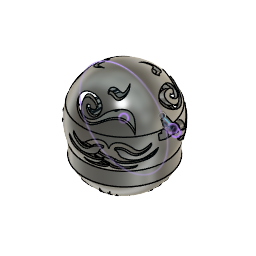
board+case (Autodesk Fusion 360 design; units mm, degrees)
part number: 2025-12-10-14-29-19-279
part number: 2025-12-10-14-29-30-996
part number: 2025-12-10-16-31-34-686
part number: 2025-12-10-16-59-24-375
part number: 2025-12-10-23-41-42-492
part number: 2025-12-11-01-50-10-497
part number: 2025-12-11-01-57-33-360
part number: 2025-12-11-03-29-09-115
Autodesk Fusion 360 part; units mm, degrees
(part 1 of 2)
sketch "Sketch1" plane through (0, 0, 0) normal (0, 0, 1) x (1, 0, 0) in component "base"
  circle A0 centre (0, 0) radius 0.45
  circle A1 centre (2.54, 0) radius 0.45
  circle A2 centre (5.08, 0) radius 0.45
  circle A3 centre (7.62, 0) radius 0.45
  circle A4 centre (10.16, 0) radius 0.45
  circle A5 centre (12.7, 0) radius 0.45
  circle A6 centre (15.24, 0) radius 0.45
  circle A7 centre (17.78, 0) radius 0.45
  circle A8 centre (20.32, 0) radius 0.45
  circle A9 centre (22.86, 0) radius 0.45
  circle A10 centre (25.4, 0) radius 0.45
  circle A11 centre (27.94, 0) radius 0.45
  circle A12 centre (30.48, 0) radius 0.45
  circle A13 centre (33.02, 0) radius 0.45
  circle A14 centre (35.56, 0) radius 0.45
  circle A15 centre (0, 2.54) radius 0.45
  circle A16 centre (2.54, 2.54) radius 0.45
  circle A17 centre (5.08, 2.54) radius 0.45
  circle A18 centre (7.62, 2.54) radius 0.45
  circle A19 centre (10.16, 2.54) radius 0.45
  circle A20 centre (12.7, 2.54) radius 0.45
  circle A21 centre (15.24, 2.54) radius 0.45
  circle A22 centre (17.78, 2.54) radius 0.45
  circle A23 centre (20.32, 2.54) radius 0.45
  circle A24 centre (22.86, 2.54) radius 0.45
  circle A25 centre (25.4, 2.54) radius 0.45
  circle A26 centre (27.94, 2.54) radius 0.45
  circle A27 centre (30.48, 2.54) radius 0.45
  circle A28 centre (33.02, 2.54) radius 0.45
  circle A29 centre (35.56, 2.54) radius 0.45
  circle A30 centre (0, 5.08) radius 0.45
  circle A31 centre (2.54, 5.08) radius 0.45
  circle A32 centre (5.08, 5.08) radius 0.45
  circle A33 centre (7.62, 5.08) radius 0.45
  circle A34 centre (10.16, 5.08) radius 0.45
  circle A35 centre (12.7, 5.08) radius 0.45
  circle A36 centre (15.24, 5.08) radius 0.45
  circle A37 centre (17.78, 5.08) radius 0.45
  circle A38 centre (20.32, 5.08) radius 0.45
  circle A39 centre (22.86, 5.08) radius 0.45
  circle A40 centre (25.4, 5.08) radius 0.45
  circle A41 centre (27.94, 5.08) radius 0.45
  circle A42 centre (30.48, 5.08) radius 0.45
  circle A43 centre (33.02, 5.08) radius 0.45
  circle A44 centre (35.56, 5.08) radius 0.45
  circle A45 centre (0, 7.62) radius 0.45
  circle A46 centre (2.54, 7.62) radius 0.45
  circle A47 centre (5.08, 7.62) radius 0.45
  circle A48 centre (7.62, 7.62) radius 0.45
  circle A49 centre (10.16, 7.62) radius 0.45
  circle A50 centre (12.7, 7.62) radius 0.45
  circle A51 centre (15.24, 7.62) radius 0.45
  circle A52 centre (17.78, 7.62) radius 0.45
  circle A53 centre (20.32, 7.62) radius 0.45
  circle A54 centre (22.86, 7.62) radius 0.45
  circle A55 centre (25.4, 7.62) radius 0.45
  circle A56 centre (27.94, 7.62) radius 0.45
  circle A57 centre (30.48, 7.62) radius 0.45
  circle A58 centre (33.02, 7.62) radius 0.45
  circle A59 centre (35.56, 7.62) radius 0.45
  circle A60 centre (0, 10.16) radius 0.45
  circle A61 centre (2.54, 10.16) radius 0.45
  circle A62 centre (5.08, 10.16) radius 0.45
  circle A63 centre (7.62, 10.16) radius 0.45
  circle A64 centre (10.16, 10.16) radius 0.45
  circle A65 centre (12.7, 10.16) radius 0.45
  circle A66 centre (15.24, 10.16) radius 0.45
  circle A67 centre (17.78, 10.16) radius 0.45
  circle A68 centre (20.32, 10.16) radius 0.45
  circle A69 centre (22.86, 10.16) radius 0.45
  circle A70 centre (25.4, 10.16) radius 0.45
  circle A71 centre (27.94, 10.16) radius 0.45
  circle A72 centre (30.48, 10.16) radius 0.45
  circle A73 centre (33.02, 10.16) radius 0.45
  circle A74 centre (35.56, 10.16) radius 0.45
  circle A75 centre (0, 12.7) radius 0.45
  circle A76 centre (2.54, 12.7) radius 0.45
  circle A77 centre (5.08, 12.7) radius 0.45
  circle A78 centre (7.62, 12.7) radius 0.45
  circle A79 centre (10.16, 12.7) radius 0.45
  circle A80 centre (12.7, 12.7) radius 0.45
  circle A81 centre (15.24, 12.7) radius 0.45
  circle A82 centre (17.78, 12.7) radius 0.45
  circle A83 centre (20.32, 12.7) radius 0.45
  circle A84 centre (22.86, 12.7) radius 0.45
  circle A85 centre (25.4, 12.7) radius 0.45
  circle A86 centre (27.94, 12.7) radius 0.45
  circle A87 centre (30.48, 12.7) radius 0.45
  circle A88 centre (33.02, 12.7) radius 0.45
  circle A89 centre (35.56, 12.7) radius 0.45
  circle A90 centre (0, 15.24) radius 0.45
  circle A91 centre (2.54, 15.24) radius 0.45
  circle A92 centre (5.08, 15.24) radius 0.45
  circle A93 centre (7.62, 15.24) radius 0.45
  circle A94 centre (10.16, 15.24) radius 0.45
  circle A95 centre (12.7, 15.24) radius 0.45
  circle A96 centre (15.24, 15.24) radius 0.45
  circle A97 centre (17.78, 15.24) radius 0.45
  circle A98 centre (20.32, 15.24) radius 0.45
  circle A99 centre (22.86, 15.24) radius 0.45
  circle A100 centre (25.4, 15.24) radius 0.45
  circle A101 centre (27.94, 15.24) radius 0.45
  circle A102 centre (30.48, 15.24) radius 0.45
  circle A103 centre (33.02, 15.24) radius 0.45
  circle A104 centre (35.56, 15.24) radius 0.45
  circle A105 centre (0, 17.78) radius 0.45
  circle A106 centre (2.54, 17.78) radius 0.45
  circle A107 centre (5.08, 17.78) radius 0.45
  circle A108 centre (7.62, 17.78) radius 0.45
  circle A109 centre (10.16, 17.78) radius 0.45
  circle A110 centre (12.7, 17.78) radius 0.45
  circle A111 centre (15.24, 17.78) radius 0.45
  circle A112 centre (17.78, 17.78) radius 0.45
  circle A113 centre (20.32, 17.78) radius 0.45
  circle A114 centre (22.86, 17.78) radius 0.45
  circle A115 centre (25.4, 17.78) radius 0.45
  circle A116 centre (27.94, 17.78) radius 0.45
  circle A117 centre (30.48, 17.78) radius 0.45
  circle A118 centre (33.02, 17.78) radius 0.45
  circle A119 centre (35.56, 17.78) radius 0.45
  circle A120 centre (0, 20.32) radius 0.45
  circle A121 centre (2.54, 20.32) radius 0.45
  circle A122 centre (5.08, 20.32) radius 0.45
  circle A123 centre (7.62, 20.32) radius 0.45
  circle A124 centre (10.16, 20.32) radius 0.45
  circle A125 centre (12.7, 20.32) radius 0.45
  circle A126 centre (15.24, 20.32) radius 0.45
  circle A127 centre (17.78, 20.32) radius 0.45
  circle A128 centre (20.32, 20.32) radius 0.45
  circle A129 centre (22.86, 20.32) radius 0.45
  circle A130 centre (25.4, 20.32) radius 0.45
  circle A131 centre (27.94, 20.32) radius 0.45
  circle A132 centre (30.48, 20.32) radius 0.45
  circle A133 centre (33.02, 20.32) radius 0.45
  circle A134 centre (35.56, 20.32) radius 0.45
  circle A135 centre (0, 22.86) radius 0.45
  circle A136 centre (2.54, 22.86) radius 0.45
  circle A137 centre (5.08, 22.86) radius 0.45
  circle A138 centre (7.62, 22.86) radius 0.45
  circle A139 centre (10.16, 22.86) radius 0.45
  circle A140 centre (12.7, 22.86) radius 0.45
  circle A141 centre (15.24, 22.86) radius 0.45
  circle A142 centre (17.78, 22.86) radius 0.45
  circle A143 centre (20.32, 22.86) radius 0.45
  circle A144 centre (22.86, 22.86) radius 0.45
  circle A145 centre (25.4, 22.86) radius 0.45
  circle A146 centre (27.94, 22.86) radius 0.45
  circle A147 centre (30.48, 22.86) radius 0.45
  circle A148 centre (33.02, 22.86) radius 0.45
  circle A149 centre (35.56, 22.86) radius 0.45
  circle A150 centre (0, 25.4) radius 0.45
  circle A151 centre (2.54, 25.4) radius 0.45
  circle A152 centre (5.08, 25.4) radius 0.45
  circle A153 centre (7.62, 25.4) radius 0.45
  circle A154 centre (10.16, 25.4) radius 0.45
  circle A155 centre (12.7, 25.4) radius 0.45
  circle A156 centre (15.24, 25.4) radius 0.45
  circle A157 centre (17.78, 25.4) radius 0.45
  circle A158 centre (20.32, 25.4) radius 0.45
  circle A159 centre (22.86, 25.4) radius 0.45
  circle A160 centre (25.4, 25.4) radius 0.45
  circle A161 centre (27.94, 25.4) radius 0.45
  circle A162 centre (30.48, 25.4) radius 0.45
  circle A163 centre (33.02, 25.4) radius 0.45
  circle A164 centre (35.56, 25.4) radius 0.45
  circle A165 centre (0, 27.94) radius 0.45
  circle A166 centre (2.54, 27.94) radius 0.45
  circle A167 centre (5.08, 27.94) radius 0.45
  circle A168 centre (7.62, 27.94) radius 0.45
  circle A169 centre (10.16, 27.94) radius 0.45
  circle A170 centre (12.7, 27.94) radius 0.45
  circle A171 centre (15.24, 27.94) radius 0.45
  circle A172 centre (17.78, 27.94) radius 0.45
  circle A173 centre (20.32, 27.94) radius 0.45
  circle A174 centre (22.86, 27.94) radius 0.45
  circle A175 centre (25.4, 27.94) radius 0.45
  circle A176 centre (27.94, 27.94) radius 0.45
  circle A177 centre (30.48, 27.94) radius 0.45
  circle A178 centre (33.02, 27.94) radius 0.45
  circle A179 centre (35.56, 27.94) radius 0.45
  circle A180 centre (0, 30.48) radius 0.45
  circle A181 centre (2.54, 30.48) radius 0.45
  circle A182 centre (5.08, 30.48) radius 0.45
  circle A183 centre (7.62, 30.48) radius 0.45
  circle A184 centre (10.16, 30.48) radius 0.45
  circle A185 centre (12.7, 30.48) radius 0.45
  circle A186 centre (15.24, 30.48) radius 0.45
  circle A187 centre (17.78, 30.48) radius 0.45
  circle A188 centre (20.32, 30.48) radius 0.45
  circle A189 centre (22.86, 30.48) radius 0.45
  circle A190 centre (25.4, 30.48) radius 0.45
  circle A191 centre (27.94, 30.48) radius 0.45
  circle A192 centre (30.48, 30.48) radius 0.45
  circle A193 centre (33.02, 30.48) radius 0.45
  circle A194 centre (35.56, 30.48) radius 0.45
  circle A195 centre (0, 33.02) radius 0.45
  circle A196 centre (2.54, 33.02) radius 0.45
  circle A197 centre (5.08, 33.02) radius 0.45
  circle A198 centre (7.62, 33.02) radius 0.45
  circle A199 centre (10.16, 33.02) radius 0.45
  circle A200 centre (12.7, 33.02) radius 0.45
  circle A201 centre (15.24, 33.02) radius 0.45
  circle A202 centre (17.78, 33.02) radius 0.45
  circle A203 centre (20.32, 33.02) radius 0.45
  circle A204 centre (22.86, 33.02) radius 0.45
  circle A205 centre (25.4, 33.02) radius 0.45
  circle A206 centre (27.94, 33.02) radius 0.45
  circle A207 centre (30.48, 33.02) radius 0.45
  circle A208 centre (33.02, 33.02) radius 0.45
  circle A209 centre (35.56, 33.02) radius 0.45
  circle A210 centre (0, 35.56) radius 0.45
  circle A211 centre (2.54, 35.56) radius 0.45
  circle A212 centre (5.08, 35.56) radius 0.45
  circle A213 centre (7.62, 35.56) radius 0.45
  circle A214 centre (10.16, 35.56) radius 0.45
  circle A215 centre (12.7, 35.56) radius 0.45
  circle A216 centre (15.24, 35.56) radius 0.45
  circle A217 centre (17.78, 35.56) radius 0.45
  circle A218 centre (20.32, 35.56) radius 0.45
  circle A219 centre (22.86, 35.56) radius 0.45
  circle A220 centre (25.4, 35.56) radius 0.45
  circle A221 centre (27.94, 35.56) radius 0.45
  circle A222 centre (30.48, 35.56) radius 0.45
  circle A223 centre (33.02, 35.56) radius 0.45
  circle A224 centre (35.56, 35.56) radius 0.45
  line L0 (-2, 38) -> (38, 38)
  line L1 (38, 38) -> (38, -2)
  line L2 (38, -2) -> (-2, -2)
  line L3 (-2, -2) -> (-2, 38)
  dimension "d1" = 0.9
  dimension "d4" = 2.54
  dimension "d5" = 2.54
  dimension "d6" = 40
  dimension "d7" = 40
  constraint coincident A0.centre origin
  constraint horizontal L0
  constraint vertical L1
  constraint horizontal L2
  constraint vertical L3
  measures "d1" diameter of A0
  measures "d6" distance of L0.start L0.end
  measures "d7" distance of L0.start L2.end
extrude "Extrude1" add sketch "Sketch1" along normal blind 2 contours A0 | A1 | A2 | A3 | A4 | A5 | A6 | A7 | A8 | A9 | A10 | A11 | A12 | A13 | A14 | A15 | A17 | A18 | A19 | A20 | A21 | A22 | A23 | A24 | A25 | A27 | A28 | A29 | A30 | A31 | A32 | A33 | A34 | A35 | A36 | A37 | A38 | A39 | A40 | A41 | A42 | A43 | A44 | A45 | A46 | A47 | A48 | A49 | A50 | A51 | A52 | A53 | A54 | A55 | A56 | A57 | A58 | A59 | A60 | A61 | A62 | A63 | A64 | A65 | A66 | A67 | A68 | A69 | A70 | A71 | A72 | A73 | A74 | A75 | A76 | A77 | A78 | A79 | A80 | A81 | A82 | A83 | A84 | A85 | A86 | A87 | A88 | A89 | A90 | A91 | A92 | A93 | A94 | A95 | A96 | A97 | A98 | A99 | A100 | A101 | A102 | A103 | A104 | A105 | A106 | A107 | A108 | A109 | A110 | A111 | A112 | A113 | A114 | A115 | A116 | A117 | A118 | A119 | A120 | A121 | A122 | A123 | A124 | A125 | A126 | A127 | A128 | A129 | A130 | A131 | A132 | A133 | A134 | A135 | A136 | A137 | A138 | A139 | A140 | A141 | A142 | A143 | A144 | A145 | A146 | A147 | A148 | A149 | A150 | A151 | A152 | A153 | A154 | A155 | A156 | A157 | A158 | A159 | A160 | A161 | A162 | A163 | A164 | A165 | A167 | A168 | A169 | A170 | A171 | A172 | A173 | A174 | A175 | A177 | A178 | A179 | A180 | A181 | A182 | A183 | A184 | A185 | A186 | A187 | A188 | A189 | A190 | A191 | A192 | A193 | A194 | A195 | A196 | A197 | A198 | A199 | A200 | A201 | A202 | A203 | A204 | A205 | A206 | A207 | A208 | A209 | A210 | A211 | A212 | A213 | A214 | A215 | A216 | A217 | A218 | A219 | A220 | A221 | A222 | A223 | A224 | L0 L1 L2 L3 makes body 1 in component "base"
sketch "Sketch2" plane through (0, 0, 0) normal (0, 0, -1) x (1, 0, 0) in component "base"
  circle A0 centre (2.54, -27.94) radius 0.45
  circle A1 centre (27.94, -2.54) radius 0.45
  circle A2 centre (27.94, -27.94) radius 0.45
  circle A3 centre (2.54, -2.54) radius 0.45
  line L0 (38, 2) -> (-2, 2)
  line L1 (-2, 2) -> (-2, -38)
  line L2 (-2, -38) -> (38, -38)
  line L3 (38, -38) -> (38, 2)
  line L4 (39.5, 3.5) -> (-3.5, 3.5)
  line L5 (-3.5, 3.5) -> (-3.5, -39.5)
  line L6 (-3.5, -39.5) -> (39.5, -39.5)
  line L7 (39.5, -39.5) -> (39.5, 3.5)
  dimension "d10" = 1.5
extrude "Extrude2" add sketch "Sketch2" against normal blind 27 contours L4 L5 L6 L7 bodies 1 in component "base"
sketch "Sketch3" plane through (0, 0, 27) normal (0, 0, 1) x (-1, 0, 0) in component "base"
  line L0 (-38, -38) -> (-38, 2)
  line L1 (-38, 2) -> (2, 2)
  line L2 (2, 2) -> (2, -38)
  line L3 (2, -38) -> (-38, -38)
  line L4 (-39.5, 3.5) -> (-39.5, -39.5)
  line L5 (-39.5, -39.5) -> (3.5, -39.5)
  line L6 (3.5, -39.5) -> (3.5, 3.5)
  line L7 (3.5, 3.5) -> (-39.5, 3.5)
sketch "Sketch4" plane through (0, 0, 0) normal (0, 0, -1) x (1, 0, 0) in component "base"
  line L0 (39.5, -39.5) -> (39.5, 3.5)
  line L1 (39.5, 3.5) -> (-3.5, 3.5)
  line L2 (-3.5, 3.5) -> (-3.5, -39.5)
  line L3 (-3.5, -39.5) -> (39.5, -39.5)
  circle A0 centre (2.54, -27.94) radius 0.45
  circle A1 centre (27.94, -2.54) radius 0.45
  circle A2 centre (27.94, -27.94) radius 0.45
  circle A3 centre (2.54, -2.54) radius 0.45
  line L4 (-3.5, -18) -> (-15.5, -18)
  line L5 (-15.5, -18) -> (-15.5, -9.5)
  line L6 (-15.5, -18) -> (-15.5, -26.5)
  line L7 (-15.5, -26.5) -> (-3.5, -26.5)
  line L8 (-15.5, -9.5) -> (-3.5, -9.5)
  line L9 (-17, -28) -> (-3.5, -28)
  line L10 (-17, -18) -> (-17, -28)
  line L11 (-17, -18) -> (-17, -8)
  line L12 (-17, -8) -> (-3.5, -8)
  dimension "d13" = 12
  dimension "d14" = 8.5
  dimension "d15" = 8.5
  dimension "d16" = 1.5
  constraint midpoint L2 L4.start
  constraint perpendicular L2 L4
  constraint perpendicular L4 L5
  constraint perpendicular L4 L6
  constraint coincident L2 L7.end
  constraint perpendicular L2 L7
  constraint coincident L2 L8.end
  constraint perpendicular L2 L8
  measures "d13" distance of L4.start L4.end
  measures "d14" distance of L4.end L5.end
  measures "d15" distance of L4.end L6.end
extrude "Extrude3" add sketch "Sketch4" against normal blind 27 contours L2 L5 L6 L7 L8 L9 L10 L11 L12 bodies 1 in component "base"
extrude "Extrude4" add sketch "Sketch4" against normal blind 2 contours L2 L4 L6 L7 | L2 L4 L5 L8 bodies 1 in component "base"
sketch "Sketch5" plane through (0, 0, 27) normal (0, 0, 1) x (-1, 0, 0) in component "base"
  line L0 (2, 2) -> (2, -38)
  line L1 (3.5, -39.5) -> (3.5, 3.5)
  line L2 (15.5, -26.5) -> (3.5, -26.5)
  line L3 (15.5, -9.5) -> (3.5, -9.5)
  line L4 (2, -26.5) -> (3.5, -26.5)
  line L5 (3.5, -9.5) -> (2, -9.5)
  line L6 (2, -26.5) -> (2, -24)
  line L7 (2, -24) -> (3.5, -24)
  line L8 (2, -9.5) -> (2, -12)
  line L9 (2, -12) -> (3.5, -12)
  line L10 (0, -38) -> (-36, -38)
  line L11 (-36, -38) -> (-36, -39.5)
  line L12 (-36, -39.5) -> (0, -39.5)
  line L13 (0, -39.5) -> (0, -38)
  line L14 (0, 2) -> (-36, 2)
  line L15 (-36, 2) -> (-36, 3.5)
  line L16 (-36, 3.5) -> (0, 3.5)
  line L17 (0, 3.5) -> (0, 2)
  dimension "d22" = 1.5
  constraint coincident L2.end L4.end
  constraint coincident L3.end L5.start
  constraint coincident L0 L5.end
  constraint perpendicular L0 L5
  constraint coincident L1 L7.end
  constraint perpendicular L1 L7
  constraint coincident L0 L8.end
  constraint coincident L1 L9.end
  constraint perpendicular L1 L9
  constraint horizontal L10
  constraint vertical L11
  constraint horizontal L12
  constraint vertical L13
  constraint horizontal L14
  constraint vertical L15
  constraint horizontal L16
  constraint vertical L17
  measures "d22" distance of L14.start L16.end
extrude "Extrude5" cut sketch "Sketch5" against normal blind 19 contours L0 L1 L7 L9 | L10 L11 L12 L13 | L14 L15 L16 L17 bodies 1 in component "base"
sketch "Sketch6" plane through (-17, 0, 0) normal (-1, 0, 0) x (0, -1, 0) in component "base"
  line L0 (-28, 0) -> (-8, 0)
  line L1 (-8, 0) -> (-8, 27)
  line L2 (-8, 27) -> (-28, 27)
  line L3 (-28, 27) -> (-28, 0)
  circle A0 centre (-18, 10) radius 8
  line L4 (-26, 10) -> (-26, 27)
  line L5 (-10, 10) -> (-10, 27)
  constraint coincident A0 L4.start
  constraint coincident L2 L4.end
  constraint tangent A0 L4
  constraint perpendicular L2 L4
  constraint coincident A0 L5.start
  constraint coincident L2 L5.end
  constraint tangent A0 L5
  constraint perpendicular L2 L5
extrude "Extrude6" cut sketch "Sketch6" against normal blind 2 contours L2 A0 L4 L5 | A0 bodies 1 in component "base"
extrude "Extrude7" cut sketch "Sketch3" 2 faces at (-2.5, 6, 27) (-2.5, 30, 27) against normal blind 6 on bodies 1 bodies 1 in component "base"
move_face "OffsetFaces1" offset 3 3 faces at (-16.5, 26, 17.3333) (-16.5, 18, 2) (-16.5, 10, 17.3333) on bodies 1 in component "base"
move_face "MoveFace1" by (6, 0, 0) 1 faces at (-15.5, 25.3333, 11) on bodies 1 in component "base"
move_face "MoveFace2" by (6, 0, 0) 1 faces at (-17, 26.3333, 10.3333) on bodies 1 in component "base"
move_face "MoveFace3" by (-4, 0, 0) 3 faces at (38, 24.6667, 14.6667) (36, -2.5, 16.6667) (36, 39, 12.3333) on bodies 1 in component "base"
move_face "MoveFace4" by (-4, 0, 0) 1 faces at (39.5, 10.8333, 14) on bodies 1 in component "base"
move_face "MoveFace5" by (0, -4, 0) 2 faces at (10.6667, 38, 4) (10.6667, 39.5, 2.6667) on bodies 1 in component "base"
move_face "OffsetFaces2" offset -0.5 1 faces at (2.9878, 2.5848, 1.3333) on bodies 1 in component "base"
move_face "OffsetFaces3" offset -0.5 1 faces at (2.156, 28.1746, 1.3333) on bodies 1 in component "base"
move_face "OffsetFaces4" offset -0.5 1 faces at (28.3352, 28.1552, 0.6667) on bodies 1 in component "base"
move_face "OffsetFaces5" offset -0.5 1 faces at (28.1453, 2.9404, 0.6667) on bodies 1 in component "base"
sketch "Sketch1 (2)" plane through (0, -3.5, 0) normal (0, -1, 0) x (1, 0, 0) in component "ball"
  line L0 (35.5, 21) -> (32, 21)
  line L1 (32, 21) -> (32, 8)
  line L2 (32, 8) -> (0, 8)
  line L3 (0, 8) -> (0, 21)
  line L4 (0, 21) -> (-3.5, 21)
  line L5 (-3.5, 21) -> (-3.5, 0)
  line L6 (-3.5, 0) -> (35.5, 0)
  line L7 (35.5, 0) -> (35.5, 21)
ref_plane "WorkPlane1" through (16, 16, 10.5) normal (0, 1, 0) x (-1, 0, 0) in component "ball"
sketch "Sketch2 (2)" plane through (0, 16, 0) normal (0, 1, 0) x (1, 0, 0) in component "ball"
  line L0 (-11, 0) -> (-11, -21)
  line L1 (35.5, 0) -> (35.5, -21)
  circle A0 centre (14.9383, -11.3653) radius 31
  circle A1 centre (14.9383, -11.3653) radius 32.5
  line L2 (39.5, 0) -> (-3.5, 0)
  line L3 (-16.0701, -21.0981) -> (45.9467, -21.0981)
  line L4 (-12.4633, 3.1313) -> (-12.4633, -21.0981)
  line L5 (14.9383, -11.3653) -> (14.9383, 21.1347)
  dimension "d34" = 62
  dimension "d35" = 1.5
  constraint coincident A1 L3.start
  constraint coincident A1 L3.end
  constraint horizontal L3
  constraint coincident A0 L4.start
  constraint coincident L3 L4.end
  constraint perpendicular L3 L4
  constraint coincident A0.centre A1.centre
  constraint parallel L1 L5
  constraint coincident A1 L5.end
  measures "d34" diameter of A0
revolve "Revolve1" add sketch "Sketch2 (2)" angle 360 about axis through (14.9383, 16, 11.3653) along (0, 0, -1) separate body contours A0 A1 L3 L5 picked at (17.9506, 20.4192) makes body 2 in component "ball"
sketch "Sketch3 (2)" plane through (0, 0, 0) normal (0, 0, -1) x (1, 0, 0) in component "ball"
  line L0 (-3.5, -28) -> (-3.5, -35.5)
  line L1 (-3.5, -35.5) -> (35.5, -35.5)
  line L2 (35.5, -35.5) -> (35.5, 3.5)
  line L3 (35.5, 3.5) -> (-3.5, 3.5)
  line L4 (-3.5, 3.5) -> (-3.5, -8)
  line L5 (-3.5, -8) -> (-11, -8)
  line L6 (-11, -8) -> (-11, -28)
  line L7 (-11, -28) -> (-3.5, -28)
  circle A0 centre (2.54, -27.94) radius 0.95
  circle A1 centre (27.94, -2.54) radius 0.95
  circle A2 centre (27.94, -27.94) radius 0.95
  circle A3 centre (2.54, -2.54) radius 0.95
  line L8 (35.5, -35.5) -> (35.5, 3.5)
  line L9 (-17, -28) -> (-3.5, -28)
  line L10 (-11, -23) -> (-11, -28)
  line L11 (-2, -12) -> (-3.5, -12)
  line L12 (-3.5, -12) -> (-3.5, -9.5)
  line L13 (-3.5, -9.5) -> (-9.5, -9.5)
  line L14 (-9.5, -9.5) -> (-9.5, -13)
  line L15 (-9.5, -13) -> (-11, -13)
  line L16 (-11, -13) -> (-11, -8)
  line L17 (-11, -8) -> (-3.5, -8)
  line L18 (-3.5, -8) -> (-3.5, 3.5)
  line L19 (-3.5, 3.5) -> (0, 3.5)
  line L20 (0, 3.5) -> (0, 2)
  line L21 (0, 2) -> (-2, 2)
  line L22 (-2, 2) -> (-2, -12)
  line L23 (-9.5, -13) -> (-9.5, -23)
  line L24 (-9.5, -23) -> (-11, -23)
  line L25 (-11, -23) -> (-11, -13)
  line L26 (-11, -13) -> (-9.5, -13)
  line L27 (0, 3.5) -> (32, 3.5)
  line L28 (32, 3.5) -> (32, 2)
  line L29 (32, 2) -> (0, 2)
  line L30 (0, 2) -> (0, 3.5)
  line L31 (32, -35.5) -> (32, -34)
  line L32 (32, -34) -> (34, -34)
  line L33 (34, -34) -> (34, 2)
  line L34 (34, 2) -> (32, 2)
  line L35 (32, 2) -> (32, 3.5)
  line L36 (32, 3.5) -> (35.5, 3.5)
  line L37 (35.5, 3.5) -> (35.5, -35.5)
  line L38 (35.5, -35.5) -> (32, -35.5)
  line L39 (0, -35.5) -> (0, -34)
  line L40 (0, -34) -> (32, -34)
  line L41 (32, -34) -> (32, -35.5)
  line L42 (32, -35.5) -> (0, -35.5)
  line L43 (-3.5, -24) -> (-2, -24)
  line L44 (-2, -24) -> (-2, -34)
  line L45 (-2, -34) -> (0, -34)
  line L46 (0, -34) -> (0, -35.5)
  line L47 (0, -35.5) -> (-3.5, -35.5)
  line L48 (-3.5, -35.5) -> (-3.5, -28)
  line L49 (-3.5, -28) -> (-11, -28)
  line L50 (-11, -28) -> (-11, -23)
  line L51 (-11, -23) -> (-9.5, -23)
  line L52 (-9.5, -23) -> (-9.5, -26.5)
  line L53 (-9.5, -26.5) -> (-3.5, -26.5)
  line L54 (-3.5, -26.5) -> (-3.5, -24)
  line L55 (-3.9, -35.9) -> (35.9, -35.9)
  line L56 (35.9, -35.9) -> (35.9, 3.9)
  line L57 (35.9, 3.9) -> (-3.9, 3.9)
  line L58 (-3.9, 3.9) -> (-3.9, -7.6)
  line L59 (-3.9, -7.6) -> (-11.4, -7.6)
  line L60 (-11.4, -7.6) -> (-11.4, -28.4)
  line L61 (-11.4, -28.4) -> (-3.9, -28.4)
  line L62 (-3.9, -28.4) -> (-3.9, -35.9)
  dimension "d42" = 0.4
extrude "Extrude1'" add sketch "Sketch3 (2)" along normal blind 1.5 separate body contours L0 L1 L6 L7 L9 L10 L24 L39 L43 L44 L45 L46 L47 L48 L49 L50 L51 L52 L53 L54 | L1 L31 L39 L40 L41 L42 L46 | L6 L15 L23 L24 L25 L26 L51 | L1 L2 L3 L8 L28 L31 L32 L33 L34 L35 L36 L37 L38 L41 | L11 L12 L13 L14 L21 L22 L23 L29 L32 L33 L34 L40 L43 L44 L45 L52 L53 L54 | L3 L4 L5 L6 L11 L12 L13 L14 L15 L16 L17 L18 L19 L20 L21 L22 L26 L30 | L3 L20 L27 L28 L29 L30 L35 | A0 | A1 | A3 | L55 L56 L57 L58 L59 L60 L61 L62 makes body 3 in component "ball"
sketch "Sketch4 (2)" plane through (0, 0, 0) normal (0, 0, 1) x (-1, 0, 0) in component "ball"
  circle A0 centre (-27.94, -27.94) radius 0.95
  line L0 (3.9, -35.9) -> (3.9, -28.4)
  line L1 (3.9, -28.4) -> (11.4, -28.4)
  line L2 (11.4, -28.4) -> (11.4, -7.6)
  line L3 (11.4, -7.6) -> (3.9, -7.6)
  line L4 (3.9, -7.6) -> (3.9, 3.9)
  line L5 (3.9, 3.9) -> (-35.9, 3.9)
  line L6 (-35.9, 3.9) -> (-35.9, -35.9)
  line L7 (-35.9, -35.9) -> (3.9, -35.9)
  circle A1 centre (-14.9383, -16) radius 31.0084
  circle A2 centre (-14.9383, -16) radius 29.4325
  line L8 (5.4, -29.9) -> (12.9, -29.9)
  line L9 (12.9, -29.9) -> (12.9, -6.1)
  line L10 (12.9, -6.1) -> (5.4, -6.1)
  line L11 (5.4, -6.1) -> (5.4, 5.4)
  line L12 (5.4, 5.4) -> (-37.4, 5.4)
  line L13 (-37.4, 5.4) -> (-37.4, -37.4)
  line L14 (-37.4, -37.4) -> (5.4, -37.4)
  line L15 (5.4, -37.4) -> (5.4, -29.9)
  dimension "d45" = 1.5
extrude "Extrude2'" add sketch "Sketch4 (2)" along normal blind 1.5 contours A2 L8 L9 L10 L11 L12 L13 L14 L15 bodies 2 3 in component "ball"
split "Split1" by plane through (0, 0, -1.5) normal (0, 0, -1) bodies 2 makes body 4 at (39.4603, 11.6761, -9.5207) in component "ball"
copy_body "Body->Comp1" bodies 4 removing the originals makes body 5 in component "bottom sphere"
sketch "Sketch5 (2)" plane through (0, 16, 0) normal (0, 1, 0) x (1, 0, 0) in component "ball"
  line L0 (44.7834, 1.5) -> (-14.9069, 1.5)
  line L1 (44.7834, 1.5) -> (-14.9069, 1.5)
  line L2 (-13.266, 1.5) -> (43.1426, 1.5)
  line L3 (-1.1858, 1.5) -> (-1.1858, 13.5)
  line L4 (-1.1858, 13.5) -> (31.8142, 13.5)
  line L5 (31.8142, 13.5) -> (31.8142, 1.4986)
  line L6 (-2.6858, 1.5) -> (-2.6858, 15)
  line L7 (-2.6858, 15) -> (33.3142, 15)
  line L8 (33.3142, 15) -> (33.3142, 1.4986)
  dimension "d48" = 12
  dimension "d49" = 33
  dimension "d50" = -1.5
  constraint coincident L0 L3.start
  constraint perpendicular L0 L3
  constraint perpendicular L3 L4
  constraint vertical L5
  measures "d48" distance of L3.start L3.end
  measures "d49" distance of L3.end L4.end
sketch "Sketch1 (3)" plane through (0, 0, -1.5) normal (0, 0, -1) x (1, 0, 0) in component "bottom sphere"
  line L0 (34.9251, 3.9) -> (-3.9, 3.9)
  line L1 (-3.9, 3.9) -> (-3.9, -7.6)
  line L2 (-3.9, -7.6) -> (-11.4, -7.6)
  line L3 (-11.4, -7.6) -> (-11.4, -26.0885)
  arc A0 (34.9251, 3.9) -> (-11.4, -26.0885) centre (14.9383, -16) ccw
  arc A1 (35.9, -34.8703) -> (35.9, 2.8703) centre (14.9383, -16) ccw
  line L4 (35.9, -34.8703) -> (35.9, 2.8703)
  circle A2 centre (14.9383, -16) radius 29.8452
  arc A3 (-10.394, -28.4) -> (34.9251, -35.9) centre (14.9383, -16) ccw
  line L5 (-10.394, -28.4) -> (-3.9, -28.4)
  line L6 (-3.9, -28.4) -> (-3.9, -35.9)
  line L7 (-3.9, -35.9) -> (34.9251, -35.9)
  circle A4 centre (27.94, -27.94) radius 0.95
  line L8 (14, -11) -> (9, -8)
  line L9 (9, -8) -> (4, -8)
  line L10 (4, -8) -> (2.5494, -7.1296)
  line L11 (2.5494, -7.1296) -> (7.5494, -7.1296)
  line L12 (7.5494, -7.1296) -> (6, -4)
  line L13 (6, -4) -> (7.5494, -4.5019)
  line L14 (7.5494, -4.5019) -> (8.6825, -6.7907)
  line L15 (8.6825, -6.7907) -> (13.5, -9.5)
  line L16 (13.5, -9.5) -> (9.725, -3.6644)
  line L17 (9.725, -3.6644) -> (4.3324, -0.6316)
  line L18 (4.3324, -0.6316) -> (2.7789, 2.5062)
  line L19 (2.7789, 2.5062) -> (4.6432, 0.2584)
  line L20 (4.6432, 0.2584) -> (9.3089, -2.148)
  line L21 (9.3089, -2.148) -> (6.0955, 4.3428)
  line L22 (6.0955, 4.3428) -> (3.7111, 6.6775)
  line L23 (3.7111, 6.6775) -> (6.6837, 5.1443)
  line L24 (6.6837, 5.1443) -> (10.1225, -1.8016)
  line L25 (10.1225, -1.8016) -> (12.5, -6)
  line L26 (12.5, -6) -> (11.3112, 2.7576)
  line L27 (11.3112, 2.7576) -> (8.4031, 9.2927)
  line L28 (8.4031, 9.2927) -> (10.5, 7.5)
  line L29 (10.5, 7.5) -> (12.102, 3.9)
  line L30 (14, -11) -> (14, -16)
  line L31 (12.102, 3.9) -> (15, -6)
  line L32 (15, -6) -> (14.9383, -16)
  line L33 (15.9382, -11.012) -> (15.8765, -16.0116)
  line L34 (15.9382, -11.012) -> (20.9749, -8.0739)
  line L35 (20.9749, -8.0739) -> (25.9745, -8.1356)
  line L36 (25.9745, -8.1356) -> (27.4357, -7.2832)
  line L37 (27.4357, -7.2832) -> (22.4361, -7.2215)
  line L38 (22.4361, -7.2215) -> (24.024, -4.1112)
  line L39 (24.024, -4.1112) -> (22.4685, -4.5939)
  line L40 (22.4685, -4.5939) -> (21.3072, -6.8686)
  line L41 (21.3072, -6.8686) -> (16.4567, -9.5182)
  line L42 (16.4567, -9.5182) -> (20.3035, -3.7297)
  line L43 (20.3035, -3.7297) -> (25.733, -0.7637)
  line L44 (25.733, -0.7637) -> (27.3251, 2.3548)
  line L45 (27.3251, 2.3548) -> (25.4333, 0.1301)
  line L46 (25.4333, 0.1301) -> (20.7382, -2.2185)
  line L47 (20.7382, -2.2185) -> (24.0315, 4.2322)
  line L48 (24.0315, 4.2322) -> (26.4445, 6.5372)
  line L49 (26.4445, 6.5372) -> (23.4532, 5.0408)
  line L50 (23.4532, 5.0408) -> (19.929, -1.8621)
  line L51 (19.929, -1.8621) -> (17.4998, -6.0309)
  line L52 (17.4998, -6.0309) -> (18.7966, 2.7114)
  line L53 (18.7966, 2.7114) -> (21.7851, 9.2101)
  line L54 (21.7851, 9.2101) -> (19.6663, 7.4434)
  line L55 (19.6663, 7.4434) -> (18.0199, 3.8635)
  line L56 (18.0199, 3.8635) -> (15, -6)
  line L57 (14, -16) -> (15.8765, -16.0116)
  line L58 (3.8458, -15.05) -> (8.5657, -17.9259)
  line L59 (5.0558, -14.7352) -> (2.6094, -10.3746)
  line L60 (2.6094, -10.3746) -> (1.1406, -9.5353)
  line L61 (10.1186, -17.6281) -> (5.0558, -14.7352)
  line L62 (0.1992, -18.7469) -> (5.024, -18.7662)
  line L63 (1.1406, -9.5353) -> (3.587, -13.896)
  line L64 (10.0907, -26.0223) -> (10.0283, -20.4956)
  line L65 (6.0057, -33.045) -> (5.7568, -27.8012)
  line L66 (-3.6541, -14.2696) -> (-7.1508, -14.4501)
  line L67 (-7.1299, -18.2411) -> (-10.3326, -17.3039)
  line L68 (-10.3326, -17.3039) -> (-7.541, -19.1463)
  line L69 (5.024, -18.7662) -> (-3.1954, -22.0144)
  line L70 (10.9508, -26.8341) -> (9.0151, -29.7408)
  line L71 (1.7423, -33.8295) -> (0.9126, -37.0618)
  line L72 (-3.1942, -31.5937) -> (-0.8775, -28.4063)
  line L73 (10.0283, -20.4956) -> (6.862, -26.6827)
  line L74 (11.0773, -19.3126) -> (10.9792, -25.1427)
  line L75 (13.4792, -29.4728) -> (13.4508, -31.1643)
  line L76 (-0.8775, -28.4063) -> (6.2472, -20.9466)
  line L77 (0.9126, -37.0618) -> (0.7541, -33.7208)
  line L78 (10.1186, -17.6281) -> (14.4792, -15.1817)
  line L79 (9.0151, -29.7408) -> (8.6751, -28.148)
  line L80 (5.05, -27.2698) -> (7.4972, -23.1116)
  line L81 (-3.8048, -23.263) -> (6.2472, -20.9466)
  line L82 (6.2472, -20.9466) -> (14.9383, -16)
  line L83 (6.9318, -32.8691) -> (4.9911, -35.7834)
  line L84 (8.6751, -28.148) -> (10.0907, -26.0223)
  line L85 (13.4508, -31.1643) -> (10.9508, -26.8341)
  line L86 (4.9911, -35.7834) -> (6.0057, -33.045)
  line L87 (0.0995, -14.0759) -> (1.2953, -15.1817)
  line L88 (-7.7283, -23.6272) -> (-3.8048, -23.263)
  line L89 (8.5657, -17.9259) -> (1.6293, -17.4888)
  line L90 (-3.1954, -22.0144) -> (-10.3177, -22.6755)
  line L91 (-7.541, -19.1463) -> (0.1992, -18.7469)
  line L92 (-7.1508, -14.4501) -> (-4.2783, -14.9761)
  line L93 (7.4972, -23.1116) -> (0.5073, -28.5199)
  line L94 (-4.2783, -14.9761) -> (0.1033, -17.8679)
  line L95 (-3.6982, -34.306) -> (-3.1942, -31.5937)
  line L96 (11.0773, -19.3126) -> (15.4074, -16.8126)
  line L97 (0.1033, -17.8679) -> (-7.1299, -18.2411)
  line L98 (6.862, -26.6827) -> (6.9318, -32.8691)
  line L99 (0.7541, -33.7208) -> (5.05, -27.2698)
  line L100 (15.4074, -16.8126) -> (14.4792, -15.1817)
  line L101 (-10.3177, -22.6755) -> (-7.7283, -23.6272)
  line L102 (0.5073, -28.5199) -> (-3.6982, -34.306)
  line L103 (5.7568, -27.8012) -> (1.7423, -33.8295)
  line L104 (10.9792, -25.1427) -> (13.4792, -29.4728)
  line L105 (3.587, -13.896) -> (0.0995, -14.0759)
  line L106 (1.2953, -15.1817) -> (3.8458, -15.05)
  line L107 (1.6293, -17.4888) -> (-3.6541, -14.2696)
  line L108 (19.6619, -26.0814) -> (19.7925, -20.5559)
  line L109 (18.7842, -25.1909) -> (16.231, -29.4898)
  line L110 (16.231, -29.4898) -> (16.2386, -31.1815)
  line L111 (18.7581, -19.36) -> (18.7842, -25.1909)
  line L112 (24.6867, -27.391) -> (22.2911, -23.2029)
  line L113 (16.2386, -31.1815) -> (18.7918, -26.8825)
  line L114 (26.0417, -15.187) -> (21.2866, -18.0044)
  line L115 (34.166, -15.2134) -> (29.7492, -18.0508)
  line L116 (22.736, -32.9667) -> (24.6406, -35.9047)
  line L117 (27.9133, -33.991) -> (28.703, -37.2333)
  line L118 (28.703, -37.2333) -> (28.9028, -33.8945)
  line L119 (22.2911, -23.2029) -> (29.2137, -28.6971)
  line L120 (26.3147, -14.0362) -> (29.7997, -14.2592)
  line L121 (36.9771, -18.5133) -> (40.1912, -17.6157)
  line L122 (37.509, -23.9063) -> (33.5903, -23.4937)
  line L123 (21.2866, -18.0044) -> (28.2279, -17.6529)
  line L124 (19.7376, -17.6874) -> (24.8356, -14.8573)
  line L125 (27.3356, -10.5272) -> (28.8147, -9.7061)
  line L126 (33.5903, -23.4937) -> (23.5677, -21.0534)
  line L127 (40.1912, -17.6157) -> (37.3771, -19.4235)
  line L128 (18.7581, -19.36) -> (14.4592, -16.8067)
  line L129 (29.7997, -14.2592) -> (28.5904, -15.3501)
  line L130 (29.6424, -18.9286) -> (24.8177, -18.8884)
  line L131 (30.5998, -28.6005) -> (23.5677, -21.0534)
  line L132 (23.5677, -21.0534) -> (14.9383, -16)
  line L133 (33.5506, -14.4992) -> (37.0448, -14.7228)
  line L134 (28.5904, -15.3501) -> (26.0417, -15.187)
  line L135 (28.8147, -9.7061) -> (26.3147, -14.0362)
  line L136 (37.0448, -14.7228) -> (34.166, -15.2134)
  line L137 (20.6914, -29.8128) -> (21.0511, -28.2244)
  line L138 (32.8769, -31.8163) -> (30.5998, -28.6005)
  line L139 (19.7925, -20.5559) -> (22.8821, -26.7815)
  line L140 (29.2137, -28.6971) -> (33.3475, -34.5346)
  line L141 (28.9028, -33.8945) -> (24.6867, -27.391)
  line L142 (24.6406, -35.9047) -> (23.6599, -33.154)
  line L143 (24.8177, -18.8884) -> (32.9964, -22.2377)
  line L144 (23.6599, -33.154) -> (23.9734, -27.9136)
  line L145 (40.11, -22.9867) -> (37.509, -23.9063)
  line L146 (19.7376, -17.6874) -> (15.4074, -15.1874)
  line L147 (23.9734, -27.9136) -> (27.9133, -33.991)
  line L148 (28.2279, -17.6529) -> (33.5506, -14.4992)
  line L149 (37.3771, -19.4235) -> (29.6424, -18.9286)
  line L150 (15.4074, -15.1874) -> (14.4592, -16.8067)
  line L151 (33.3475, -34.5346) -> (32.8769, -31.8163)
  line L152 (32.9964, -22.2377) -> (40.11, -22.9867)
  line L153 (29.7492, -18.0508) -> (36.9771, -18.5133)
  line L154 (24.8356, -14.8573) -> (27.3356, -10.5272)
  line L155 (18.7918, -26.8825) -> (20.6914, -29.8128)
  line L156 (21.0511, -28.2244) -> (19.6619, -26.0814)
  line L157 (22.8821, -26.7815) -> (22.736, -32.9667)
  circle A5 centre (14.9383, -16) radius 2.5
  point P0 (8.551, -36.9369)
  point P1 (14.9383, -16)
  point P2 (14.9383, -16)
  point P3 (36.2638, -11.0631)
  point P4 (14.9383, -16)
  point P5 (14.9383, -16)
  dimension "d52" = 360
  dimension "d61" = 5
  constraint horizontal L9
  constraint parallel L8 L10
  constraint parallel L9 L11
  constraint parallel L12 L14
  constraint parallel L15 L17
  constraint parallel L12 L18
  constraint parallel L18 L21
  constraint parallel L20 L23
  constraint parallel L21 L24
  constraint coincident L0 L29.end
  constraint parallel L27 L29
  constraint vertical L30
  constraint coincident P5 P4
  constraint symmetric L8.start L32 L33.start
  constraint symmetric L8.end L32 L34.end
  constraint symmetric L9.end L32 L35.end
  constraint symmetric L10.end L32 L36.end
  constraint symmetric L11.end L32 L37.end
  constraint symmetric L12.end L32 L38.end
  constraint symmetric L13.end L32 L39.end
  constraint symmetric L14.end L32 L40.end
  constraint symmetric L15.end L32 L41.end
  constraint symmetric L16.end L32 L42.end
  constraint symmetric L17.end L32 L43.end
  constraint symmetric L18.end L32 L44.end
  constraint symmetric L19.end L32 L45.end
  constraint symmetric L20.end L32 L46.end
  constraint symmetric L21.end L32 L47.end
  constraint symmetric L22.end L32 L48.end
  constraint symmetric L23.end L32 L49.end
  constraint symmetric L24.end L32 L50.end
  constraint symmetric L25.end L32 L51.end
  constraint symmetric L26.end L32 L52.end
  constraint symmetric L27.end L32 L53.end
  constraint symmetric L28.end L32 L54.end
  constraint symmetric L29.end L32 L55.end
  constraint symmetric L30.end L32 L33.end
  constraint symmetric L31.end L32 L56.end
  constraint concentric A1 A5
  measures "d61" diameter of A5
extrude "Extrude1''" cut sketch "Sketch1 (3)" along normal blind 29 contours L0 L32 L33 L34 L35 L36 L37 L38 L39 L40 L41 L42 L43 L44 L45 L46 L47 L50 L51 L52 L53 L55 L56 A5 | L0 L47 L48 L49 L50 | L0 L53 L54 L55 | L0 L8 L9 L10 L11 L12 L13 L14 L15 L16 L17 L18 L19 L20 L21 L24 L25 L26 L27 L30 L31 L32 A5 | L0 L27 L28 L29 | L0 L21 L22 L23 L24 | L58 L59 L60 L61 L62 L63 L66 L67 L68 L69 L78 L81 L82 L87 L88 L89 L90 L91 L92 L94 L97 L101 L105 L106 L107 A5 | L4 L114 L115 L120 L122 L123 L124 L125 L126 L129 L130 L132 L133 L134 L135 L136 L143 L146 L148 L149 L152 L153 L154 A5 | L7 A4 L108 L109 L110 L111 L112 L113 L116 L117 L118 L119 L128 L131 L132 L137 L138 L139 L140 L141 L142 L144 L147 L151 L155 L156 L157 A5 | L7 L64 L65 L70 L71 L72 L73 L74 L75 L76 L77 L79 L80 L82 L83 L84 L85 L86 L93 L95 L96 L98 L99 L102 L103 L104 A5 | L4 L122 L145 L152 | L4 L121 L127 L149 L153 | L4 L133 L136 | A4 L119 | L7 L71 L77 | L7 L117 L118 picked at (27.8972, -27.5453) bodies 5 in component "bottom sphere"
sketch "Sketch2 (3)" plane through (0, 0, -1.5) normal (0, 0, 1) x (-1, 0, 0) in component "bottom sphere"
  circle A0 centre (-14.9383, -16) radius 29.8452
  circle A1 centre (-14.9383, -16) radius 28.2043
  line L0 (-44.7834, -16) -> (14.9069, -16)
  line L1 (13.266, -16) -> (13.266, -18)
  line L2 (13.266, -16) -> (13.266, -14)
  arc A2 (13.266, -14) -> (13.266, -18) centre (12.2071, -16) ccw
  line L3 (-14.9383, -16) -> (-14.9383, -18.4625)
  arc A3 (-43.1426, -18) -> (-43.1426, -14) centre (-42.0837, -16) ccw
  circle A4 centre (12.2071, -16) radius 1
  circle A5 centre (-42.0837, -16) radius 1
  dimension "d55" = 2
  dimension "d56" = 2
  dimension "d57" = 2
  dimension "d58" = 2
  constraint coincident A1 L1.start
  constraint coincident L0 L1.start
  constraint perpendicular L0 L1
  constraint tangent A1 L2
  constraint coincident A0.centre A1.centre
  constraint perpendicular L0 L3
  constraint symmetric L1.end L3 A3.start
  constraint symmetric L2.end L3 A3.end
  constraint symmetric A2 L3 A3
  constraint concentric A2 A4
  constraint concentric A3 A5
  measures "d55" distance of L1.start L1.end
  measures "d56" distance of L1.start L2.end
  measures "d57" diameter of A4
  measures "d58" diameter of A5
extrude "Extrude2''" add sketch "Sketch2 (3)" against normal blind 3 contours A1 L0 A2 A4 | A1 L0 A2 A4 | A1 L0 A3 A5 | A1 L0 A3 A5 bodies 5 in component "bottom sphere"
sketch "Sketch6 (2)" plane through (0, 0, -1.5) normal (0, 0, -1) x (1, 0, 0) in component "ball"
  line L0 (34.9251, 3.9) -> (-3.9, 3.9)
  line L1 (-3.9, 3.9) -> (-3.9, -7.6)
  line L2 (-3.9, -7.6) -> (-11.4, -7.6)
  line L3 (-11.4, -7.6) -> (-11.4, -26.0885)
  arc A0 (34.9251, 3.9) -> (-11.4, -26.0885) centre (14.9383, -16) ccw
  arc A1 (35.9, -34.8703) -> (35.9, 2.8703) centre (14.9383, -16) ccw
  line L4 (35.9, -34.8703) -> (35.9, 2.8703)
  circle A2 centre (14.9383, -16) radius 29.8452
  arc A3 (-10.394, -28.4) -> (34.9251, -35.9) centre (14.9383, -16) ccw
  line L5 (-10.394, -28.4) -> (-3.9, -28.4)
  line L6 (-3.9, -28.4) -> (-3.9, -35.9)
  line L7 (-3.9, -35.9) -> (34.9251, -35.9)
  circle A4 centre (27.94, -27.94) radius 0.95
  arc A5 (43.0689, -13.9627) -> (43.0689, -18.0373) centre (42.0837, -16) ccw
  circle A6 centre (42.0837, -16) radius 2.263
  circle A7 centre (42.0837, -16) radius 1
  circle A8 centre (42.0837, -16) radius 1
  circle A9 centre (-12.2071, -16) radius 1
  circle A10 centre (14.9383, -16) radius 29.8452
  arc A11 (43.0689, -13.9627) -> (-13.1923, -13.9627) centre (14.9383, -16) ccw
  arc A12 (-13.1923, -18.0373) -> (-13.1923, -13.9627) centre (-12.2071, -16) ccw
  arc A13 (-13.1923, -18.0373) -> (43.0689, -18.0373) centre (14.9383, -16) ccw
  arc A14 (43.0689, -13.9627) -> (43.0689, -18.0373) centre (42.0837, -16) ccw
  circle A15 centre (-12.2071, -16) radius 2.263
  circle A16 centre (-12.2071, -16) radius 1
  dimension "d62" = 2
  dimension "d65" = 2
  constraint concentric A5 A6
  constraint concentric A5 A7
  constraint concentric A9 A15
  constraint concentric A9 A16
  measures "d62" diameter of A7
  measures "d65" diameter of A16
extrude "Extrude3'" add sketch "Sketch6 (2)" against normal blind 4 contours A1 A6 | A1 A5 A6 A14 bodies 2 in component "ball"
extrude "Extrude4'" add 3 faces at (8.6589, 36.9, 0) (36.2384, 22.2258, 0) (8.6589, -4.9, 0) along direction (0, 0, -1) blind 1.5 on bodies 2 bodies 2 in component "ball"
ref_plane "WorkPlane2" through (-20, 16, 11.5) normal (-1, 0, 0) x (0, -1, 0) in component "ball"